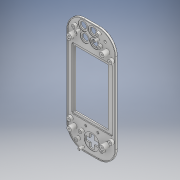
# Autodesk Inventor part: Partie Haute
Saved by Autodesk Inventor 2019 (Build 230136000, 136)
## iProperties
Created: 2018-06-04
Part Number: Partie Haute
Material: Plastique ABS
Document SubType Name: Modeling
Designer: dimercur
Mass: 33.4768 g
Surface Area: 274.719 cm^2
Volume: 31.5819 cm^3
Density: 1.06 g/cm^3
Appearance: Lisse - Blanc
Author: dimercur
Autodesk Inventor part; units mm, degrees
ref_plane "YZ Plane" through (0, 0, 0) normal (1, 0, 0) x (0, 1, 0)
ref_plane "XZ Plane" through (0, 0, 0) normal (0, 1, 0) x (-1, 0, 0)
ref_plane "XY Plane" through (0, 0, 0) normal (0, 0, 1) x (1, 0, 0)
sketch "Esquisse1" plane through (0, 0, 0) normal (0, 1, 0) x (-1, 0, 0)
  line L0 (42.5, 100) -> (-42.5, 100)
  line L1 (-42.5, 100) -> (-42.5, -100)
  line L2 (-42.5, -100) -> (42.5, -100)
  line L3 (42.5, -100) -> (42.5, 100)
  point P0 (0, 0)
  dimension "d0" = 200
  dimension "d1" = 85
  dimension "d2" = 42.5
  dimension "d3" = 100
  constraints: 8 end point, 2 parallel, 1 horizontal, 1 perpendicular
  measures "d0" distance of L2.end L0.start
  measures "d1" distance of L0.start L0.end
  measures "d2" horizontal distance of point (0, 0) L0.start
  measures "d3" vertical distance of point (0, 0) L0.start
extrude "Extrusion1" add sketch "Esquisse1" along normal blind 42
chamfer "Chanfrein1" distance 20 angle 60 1 edges at (0, 0, 100) measured on face at (0, 0.5, 100)
chamfer "Chanfrein2" distance 20 angle 60 1 edges at (0, 0, -100) measured on face at (0, 0.5, -100)
fillet "Congé3" radius 30 4 edges at (-42.5, 31, 100) (42.5, 31, 100) (-42.5, 31, -100) (42.5, 31, -100)
fillet "Congé4" radius 15 14 edges at (0, 0, 65.359) (-33.7132, 14.9269, 91.2132) (-42.5, 1.3397, 67.6795) (33.7132, 14.9269, 91.2132) (42.5, 1.3397, 67.6795) (0, 20, 100) (-42.5, 0, 0) (42.5, 0, 0) (0, 0, -65.359) (33.7132, 14.9269, -91.2132) (42.5, 1.3397, -67.6795) (-33.7132, 14.9269, -91.2132) (-42.5, 1.3397, -67.6795) (0, 20, -100)
shell "Coque1" thickness 2.5 removed faces 1 at (-14.1667, 42, -23.3333)
sketch "Esquisse3" plane through (0, 42, 0) normal (0, 1, 0) x (1, 0, 0)
  arc A0 (42.5, 70) -> (12.5, 100) centre (12.5, 70) ccw projected
  line L0 (12.5, 100) -> (-12.5, 100) projected
  arc A1 (-12.5, 100) -> (-42.5, 70) centre (-12.5, 70) ccw projected
  line L1 (-42.5, 70) -> (-42.5, -70) projected
  arc A2 (-42.5, -70) -> (-12.5, -100) centre (-12.5, -70) ccw projected
  line L2 (-12.5, -100) -> (12.5, -100) projected
  arc A3 (12.5, -100) -> (42.5, -70) centre (12.5, -70) ccw projected
  line L3 (42.5, -70) -> (42.5, 70) projected
  point P0 (0, 0)
extrude "Extrusion2" add sketch "Esquisse3" along normal blind 2.5
sketch "Esquisse4" plane through (0, 44.5, 0) normal (0, 1, 0) x (1, 0, 0)
  line L0 (36.5, 54) -> (-34.5, 54)
  line L1 (-34.5, 54) -> (-34.5, -54)
  line L2 (-34.5, -54) -> (36.5, -54)
  line L3 (36.5, -54) -> (36.5, 54)
  line L4 (27.5, -67.5897) -> (-27.5, -67.5897) projected
  line L5 (42.5, -70) -> (42.5, 70) projected
  line L6 (-42.5, 70) -> (-42.5, -70) projected
  line L7 (12.5, 100) -> (-12.5, 100) projected
  line L8 (-12.5, -100) -> (12.5, -100) projected
  point P0 (0, 0)
  dimension "d19" = 108
  dimension "d20" = 71
  dimension "d21" = 36.5
  dimension "d22" = 54
  dimension "d154" = 85
  dimension "d155" = 46
  constraints: 8 end point, 2 parallel, 1 horizontal, 1 perpendicular
  measures "d19" distance of L2.end L0.start
  measures "d20" distance of L0.start L0.end
  measures "d21" horizontal distance of point (0, 0) L0.start
  measures "d22" vertical distance of point (0, 0) L0.start
  measures "d154" distance between parallel lines of L6 L5
  measures "d155" distance between parallel lines of L8 L2
extrude "Extrusion15" cut sketch "Esquisse4" against normal through all
sketch "Esquisse5" plane through (-40, 15, 61.3397) normal (1, 0, 0) x (0, 0, -1)
  line L0 (-48.6603, 26) -> (171.3397, 26)
  line L1 (171.3397, 26) -> (171.3397, -24)
  line L2 (171.3397, -24) -> (-48.6603, -24)
  line L3 (-48.6603, -24) -> (-48.6603, 26)
  line L4 (-36.1603, 27) -> (-8.6603, 27) projected
  line L5 (-38.6603, 29.5) -> (-38.6603, 13.6603) projected
  line L6 (161.3397, 13.6603) -> (161.3397, 29.5) projected
  point P0 (61.3397, -15)
  dimension "d47" = 1
  dimension "d48" = 220
  dimension "d50" = 200
  dimension "d51" = 10
  dimension "d52" = 50
  constraints: 8 end point, 2 parallel, 1 horizontal, 1 perpendicular
  measures "d47" distance between parallel lines of L4 L0
  measures "d48" distance between parallel lines of L1 L3
  measures "d50" distance between parallel lines of L6 L5
  measures "d51" distance between parallel lines of L5 L3
  measures "d52" distance between parallel lines of L0 L2
extrude "Extrusion4" cut sketch "Esquisse5" along normal through all both and the other way through all
sketch "Esquisse6" plane through (-12.5, 41, -100) normal (0, -1, 0) x (1, 0, 0)
  line L0 (-27.5, 170) -> (-27.5, 30) projected
  arc A0 (-27.5, 30) -> (0, 2.5) centre (0, 30) ccw projected
  line L1 (0, 2.5) -> (25, 2.5) projected
  arc A1 (25, 2.5) -> (52.5, 30) centre (25, 30) ccw projected
  line L2 (52.5, 30) -> (52.5, 170) projected
  arc A2 (52.5, 170) -> (25, 197.5) centre (25, 170) ccw projected
  line L3 (25, 197.5) -> (0, 197.5) projected
  arc A3 (0, 197.5) -> (-27.5, 170) centre (0, 170) ccw projected
  line L4 (-28.75, 30) -> (-28.75, 170)
  arc A4 (0, 198.75) -> (-28.75, 170) centre (0, 170) ccw
  line L5 (0, 198.75) -> (25, 198.75)
  arc A5 (53.75, 170) -> (25, 198.75) centre (25, 170) ccw
  line L6 (53.75, 170) -> (53.75, 30)
  arc A6 (25, 1.25) -> (53.75, 30) centre (25, 30) ccw
  line L7 (25, 1.25) -> (0, 1.25)
  arc A7 (-28.75, 30) -> (0, 1.25) centre (0, 30) ccw
  line L8 (-30, 30) -> (-30, 170) projected
  point P0 (12.5, 100)
  dimension "d55" = 2.5
  dimension "d56" = 1.25
  constraints: 8 end point, 8 point on circle, 4 centre point, 7 other
  measures "d55" distance between parallel lines of L0 L8
  measures "d56" distance between parallel lines of L0 L4
extrude "Extrusion5" cut sketch "Esquisse6" against normal blind 1
sketch "Esquisse7" plane through (0, 42, 0) normal (0, -1, 0) x (1, 0, 0)
  circle A0 centre (-36, -61) radius 3.75
  circle A1 centre (36, -61) radius 3.75
  circle A2 centre (36, 61) radius 3.75
  circle A3 centre (-36, 61) radius 3.75
  point P0 (0, 0)
  dimension "d59" = 7.5
  dimension "d60" = 7.5
  dimension "d61" = 7.5
  dimension "d62" = 7.5
  dimension "d63" = 122
  dimension "d64" = 72
  dimension "d65" = 122
  dimension "d66" = 72
  dimension "d67" = 61
  dimension "d68" = 36
  dimension "d69" = 36
  dimension "d70" = 61
  constraints: 4 centre point
  measures "d59" diameter of A0
  measures "d60" diameter of A1
  measures "d61" diameter of A2
  measures "d62" diameter of A3
  measures "d63" distance of A3.centre A0.centre
  measures "d64" distance of A1.centre A0.centre
  measures "d65" distance of A2.centre A1.centre
  measures "d66" distance of A2.centre A3.centre
  measures "d67" vertical distance of point (0, 0) A0.centre
  measures "d68" horizontal distance of point (0, 0) A3.centre
  measures "d69" horizontal distance of point (0, 0) A0.centre
  measures "d70" vertical distance of point (0, 0) A1.centre
extrude "Extrusion6" add sketch "Esquisse7" along normal blind 4.5
sketch "Esquisse8" plane through (-36, 37.5, -61) normal (0, -1, 0) x (1, 0, 0)
  circle A0 centre (0, 0) radius 1.2
  circle A1 centre (0, 122) radius 1.2
  circle A2 centre (72, 122) radius 1.2
  circle A3 centre (72, 0) radius 1.2
  circle A4 centre (72, 122) radius 3.75 projected
  circle A5 centre (0, 122) radius 3.75 projected
  circle A6 centre (0, 0) radius 3.75 projected
  point P0 (36, 61)
  dimension "d73" = 2.4
  dimension "d74" = 2.4
  dimension "d75" = 2.4
  dimension "d76" = 2.4
  dimension "d77" = 72
  dimension "d78" = 122
  dimension "d79" = 122
  dimension "d80" = 72
  dimension "d81" = 122
  dimension "d82" = 72
  dimension "d83" = 61
  dimension "d84" = 61
  dimension "d85" = 36
  dimension "d86" = 36
  constraints: 4 centre point
  measures "d73" diameter of A0
  measures "d74" diameter of A1
  measures "d75" diameter of A2
  measures "d76" diameter of A3
  measures "d77" distance of A4.centre A5.centre
  measures "d78" distance of A5.centre A6.centre
  measures "d79" distance of A1.centre A0.centre
  measures "d80" distance of A2.centre A1.centre
  measures "d81" distance of A3.centre A2.centre
  measures "d82" distance of A3.centre A0.centre
  measures "d83" vertical distance of point (36, 61) A3.centre
  measures "d84" vertical distance of point (36, 61) A0.centre
  measures "d85" horizontal distance of point (36, 61) A0.centre
  measures "d86" horizontal distance of point (36, 61) A1.centre
extrude "Extrusion7" cut sketch "Esquisse8" against normal blind 5 contours A0 | A1 | A2 | A3
fillet "Congé6" radius 0.5 8 edges at (33.7132, 44.5, -91.2132) (0, 44.5, -100) (-33.7132, 44.5, -91.2132) (-42.5, 44.5, 0) (-33.7132, 44.5, 91.2132) (0, 44.5, 100) (33.7132, 44.5, 91.2132) (42.5, 44.5, 0)
sketch "Esquisse11" plane through (0, 42, 0) normal (0, -1, 0) x (1, 0, 0)
  circle A0 centre (-29.5, -70) radius 4
  circle A1 centre (27.5, -70) radius 4
  circle A2 centre (27.5, 70) radius 4
  circle A3 centre (-29.5, 70) radius 4
  line L0 (-42.5, -70) -> (-42.5, 70) projected
  line L1 (42.5, 70) -> (42.5, -70) projected
  line L2 (12.5, -100) -> (-12.5, -100) projected
  line L3 (-12.5, 100) -> (12.5, 100) projected
  circle A4 centre (-29.5, -70) radius 1.25
  circle A5 centre (27.5, -70) radius 1.25
  circle A6 centre (27.5, 70) radius 1.25
  circle A7 centre (-29.5, 70) radius 1.25
  point P0 (0, 0)
  dimension "d134" = 8
  dimension "d135" = 8
  dimension "d136" = 8
  dimension "d137" = 8
  dimension "d138" = 13
  dimension "d139" = 15
  dimension "d140" = 15
  dimension "d141" = 13
  dimension "d142" = 30
  dimension "d143" = 30
  dimension "d144" = 30
  dimension "d145" = 30
  dimension "d146" = 2.5
  dimension "d147" = 2.5
  dimension "d148" = 2.5
  dimension "d149" = 2.5
  constraints: 8 centre point, 4 coincident
  measures "d134" diameter of A0
  measures "d135" diameter of A1
  measures "d136" diameter of A3
  measures "d137" diameter of A2
  measures "d138" distance from line of L0 A0.centre
  measures "d139" distance from line of L1 A1.centre
  measures "d140" distance from line of L1 A2.centre
  measures "d141" distance from line of L0 A3.centre
  measures "d142" distance from line of A0.centre L2
  measures "d143" distance from line of L2 A1.centre
  measures "d144" distance from line of L3 A2.centre
  measures "d145" distance from line of L3 A3.centre
  measures "d146" diameter of A4
  measures "d147" diameter of A5
  measures "d148" diameter of A7
  measures "d149" diameter of A6
extrude "Extrusion10" add sketch "Esquisse11" along normal blind 10
sketch "Esquisse15" plane through (0, 44.5, 0) normal (0, 1, 0) x (1, 0, 0)
  circle A0 centre (10.5, 62) radius 0.75
  line L0 (-34.5, 54) -> (36.5, 54) projected
  line L1 (42.5, -70) -> (42.5, 70) projected
  circle A1 centre (10.5, 59) radius 0.75
  circle A2 centre (12, 60.5) radius 0.75
  circle A3 centre (9, 60.5) radius 0.75
  circle A4 centre (-10.5, 62) radius 0.75
  circle A5 centre (-10.5, 59) radius 0.75
  circle A6 centre (-9, 60.5) radius 0.75
  circle A7 centre (-12, 60.5) radius 0.75
  point P0 (0, 0)
  dimension "d189" = 1.5
  dimension "d190" = 8
  dimension "d191" = 32
  dimension "d192" = 1.5
  dimension "d193" = 1.5
  dimension "d194" = 1.5
  dimension "d195" = 32
  dimension "d196" = 5
  dimension "d197" = 6.5
  dimension "d198" = 6.5
  dimension "d199" = 3
  dimension "d200" = 3
  dimension "d201" = 30.5
  dimension "d204" = 21
  constraints: 8 centre point, 1 horizontal, 8 other
  measures "d189" diameter of A0
  measures "d190" distance from line of L0 A0.centre
  measures "d191" distance from line of L1 A0.centre
  measures "d192" diameter of A2
  measures "d193" diameter of A1
  measures "d194" diameter of A3
  measures "d195" distance from line of L1 A1.centre
  measures "d196" distance from line of L0 A1.centre
  measures "d197" distance from line of L0 A2.centre
  measures "d198" distance from line of L0 A3.centre
  measures "d199" distance of A0.centre A1.centre
  measures "d200" distance of A3.centre A2.centre
  measures "d201" distance from line of L1 A2.centre
  measures "d204" distance of A0.centre A4.centre
extrude "Extrusion13" cut sketch "Esquisse15" against normal through all
sketch "Esquisse16" plane through (0, 44.5, 0) normal (0, 1, 0) x (1, 0, 0)
  line L0 (40, 57.5) -> (-38, 57.5)
  line L1 (-38, 57.5) -> (-38, -57.5)
  line L2 (-38, -57.5) -> (40, -57.5)
  line L3 (40, -57.5) -> (40, 57.5)
  line L4 (27, 49.5) -> (-31, 49.5)
  line L5 (-31, 49.5) -> (-31, -49.5)
  line L6 (-31, -49.5) -> (27, -49.5)
  line L7 (27, -49.5) -> (27, 49.5)
  line L8 (36.5, 54) -> (36.5, -54) projected
  line L9 (-34.5, 54) -> (36.5, 54) projected
  line L10 (36.5, -54) -> (-34.5, -54) projected
  line L11 (-34.5, -54) -> (-34.5, 54) projected
  point P0 (0, 0)
  dimension "d211" = 99
  dimension "d212" = 49.5
  dimension "d213" = 78
  dimension "d215" = 3.5
  dimension "d217" = 3.5
  dimension "d218" = 3.5
  dimension "d219" = 58
  dimension "d225" = 3.5
  constraints: 16 end point, 4 parallel, 2 horizontal, 2 perpendicular
  measures "d211" distance of L6.end L4.start
  measures "d212" vertical distance of point (0, 0) L4.start
  measures "d213" distance of L0.start L0.end
  measures "d215" distance between parallel lines of L8 L3
  measures "d217" distance between parallel lines of L9 L0
  measures "d218" distance between parallel lines of L10 L2
  measures "d219" distance of L4.start L4.end
  measures "d225" distance between parallel lines of L11 L5
extrude "Extrusion14" add sketch "Esquisse16" along normal blind 1.5 and the other way blind 1 contours L3 L2 L1 L0 | L8 L10 L11 L9
chamfer "Chanfrein4" distance 0.5 angle 45 4 edges at (27, 46, 0) (-2, 46, -49.5) (-2, 46, 49.5) (-31, 46, 0)
fillet "Congé14" radius 8 4 edges at (-38, 45.25, -57.5) (-38, 45.25, 57.5) (40, 45.25, 57.5) (40, 45.25, -57.5)
fillet "Congé15" radius 0.5 16 edges at (37.6569, 44.5, -55.1569) (40, 44.5, 0) (37.6569, 44.5, 55.1569) (1, 44.5, 57.5) (-35.6569, 44.5, 55.1569) (-38, 44.5, 0) (-35.6569, 44.5, -55.1569) (1, 44.5, -57.5) (1, 46, -57.5) (37.6569, 46, -55.1569) (40, 46, 0) (37.6569, 46, 55.1569) (1, 46, 57.5) (-35.6569, 46, 55.1569) (-38, 46, 0) (-35.6569, 46, -55.1569)
fillet "Congé16" radius 3 4 edges at (36.5, 42.75, -54) (-34.5, 42.75, -54) (-34.5, 42.75, 54) (36.5, 42.75, 54)
fillet "Congé17" radius 0.5 8 edges at (35.6213, 43.5, -53.1213) (1, 43.5, -54) (-33.6213, 43.5, -53.1213) (-34.5, 43.5, 0) (-33.6213, 43.5, 53.1213) (1, 43.5, 54) (35.6213, 43.5, 53.1213) (36.5, 43.5, 0)
sketch "Esquisse9" plane through (0, 44.5, 0) normal (0, 1, 0) x (1, 0, 0)
  line L0 (10.75, 83) -> (-10.75, 83)
  line L1 (-10.75, 83) -> (-10.75, 75.5)
  line L2 (-10.75, 75.5) -> (10.75, 75.5)
  line L3 (10.75, 75.5) -> (10.75, 83)
  line L4 (3.75, 90) -> (-3.75, 90)
  line L5 (-3.75, 90) -> (-3.75, 68.5)
  line L6 (-3.75, 68.5) -> (3.75, 68.5)
  line L7 (3.75, 68.5) -> (3.75, 90)
  line L8 (12.5, 100) -> (-12.5, 100) projected
  line L9 (-42.5, 70) -> (-42.5, -70) projected
  line L10 (42.5, -70) -> (42.5, 70) projected
  point P0 (0, 0)
  dimension "d98" = 21.5
  dimension "d99" = 21.5
  dimension "d100" = 7.5
  dimension "d101" = 7.5
  dimension "d102" = 7
  dimension "d103" = 7
  dimension "d104" = 10
  dimension "d105" = 31.75
  dimension "d156" = 85
  constraints: 16 end point, 4 parallel, 2 horizontal, 2 perpendicular
  measures "d98" distance of L6.end L4.start
  measures "d99" distance of L0.start L0.end
  measures "d100" distance of L4.start L4.end
  measures "d101" distance of L2.end L0.start
  measures "d102" distance between parallel lines of L3 L7
  measures "d103" distance from line of L0 L4.start
  measures "d104" distance between parallel lines of L8 L4
  measures "d105" distance between parallel lines of L9 L1
  measures "d156" distance between parallel lines of L9 L10
extrude "Extrusion8" cut sketch "Esquisse9" against normal through all
sketch "Esquisse14" plane through (0, 44.5, 0) normal (0, 1, 0) x (1, 0, 0)
  circle A0 centre (23.25, -83) radius 2.1
  line L0 (-12.5, -100) -> (12.5, -100) projected
  line L1 (42.5, -70) -> (42.5, 70) projected
  circle A1 centre (2, -88) radius 5.5
  circle A2 centre (5, -71.2668) radius 5.5
  circle A3 centre (-12, -71.2668) radius 5.5
  circle A4 centre (-15, -88) radius 5.5
  point P0 (0, 0)
  dimension "d184" = 4.2
  dimension "d185" = 17
  dimension "d186" = 19.25
  dimension "d241" = 11
  dimension "d242" = 11
  dimension "d243" = 11
  dimension "d244" = 11
  dimension "d245" = 17
  dimension "d246" = 17
  dimension "d247" = 28
  dimension "d248" = 28
  dimension "d249" = 2
  dimension "d250" = 12
  dimension "d251" = 12
  dimension "d252" = 5
  constraints: 5 centre point
  measures "d184" diameter of A0
  measures "d185" distance from line of L0 A0.centre
  measures "d186" distance from line of L1 A0.centre
  measures "d241" diameter of A2
  measures "d242" diameter of A1
  measures "d243" diameter of A3
  measures "d244" diameter of A4
  measures "d245" distance of A4.centre A1.centre
  measures "d246" distance of A3.centre A2.centre
  measures "d249" horizontal distance of point (0, 0) A1.centre
  measures "d250" distance from line of L0 A1.centre
  measures "d251" distance from line of L0 A4.centre
  measures "d252" horizontal distance of point (0, 0) A2.centre
extrude "Extrusion12" cut sketch "Esquisse14" against normal through all
sketch "Esquisse12" plane through (0, 42, 0) normal (0, -1, 0) x (1, 0, 0)
  circle A0 centre (21.5, -81.5) radius 3
  circle A1 centre (-22.5, -85) radius 3
  line L0 (12.5, -98.75) -> (-12.5, -98.75) projected
  line L1 (-41.25, -70) -> (-41.25, 70) projected
  line L2 (41.25, 70) -> (41.25, -70) projected
  circle A2 centre (-22.5, -85) radius 1
  circle A3 centre (21.5, -81.5) radius 1
  line L3 (-12.5, 98.75) -> (12.5, 98.75) projected
  circle A4 centre (-16, -70) radius 3
  circle A5 centre (-16, -70) radius 1
  line L4 (-42.5, -70) -> (-42.5, 70) projected
  line L5 (42.5, 70) -> (42.5, -70) projected
  line L6 (12.5, -100) -> (-12.5, -100) projected
  point P0 (0, 0)
  dimension "d157" = 6
  dimension "d158" = 6
  dimension "d166" = 2
  dimension "d167" = 2
  dimension "d288" = 6
  dimension "d289" = 2
  dimension "d306" = 26.5
  dimension "d307" = 20
  dimension "d308" = 21
  dimension "d309" = 18.5
  dimension "d310" = 15
  dimension "d311" = 30
  constraints: 6 centre point, 3 coincident
  measures "d157" diameter of A1
  measures "d158" diameter of A0
  measures "d166" diameter of A2
  measures "d167" diameter of A3
  measures "d288" diameter of A4
  measures "d289" diameter of A5
  measures "d306" distance from line of A4.centre L4
  measures "d307" distance from line of A2.centre L4
  measures "d308" distance from line of A0.centre L5
  measures "d309" distance from line of L6 A0.centre
  measures "d310" distance from line of A1.centre L6
  measures "d311" distance from line of L6 A4.centre
extrude "Extrusion11" add sketch "Esquisse12" along normal blind 4.7
sketch "Esquisse17" plane through (0, 42, 0) normal (0, -1, 0) x (1, 0, 0)
  circle A0 centre (-14.769, -94.179) radius 2
  line L0 (3.75, -90) -> (-3.75, -90) projected
  line L1 (-3.75, -90) -> (-3.75, -83) projected
  point P0 (0, 0)
  dimension "d253" = 4
  dimension "d254" = 4.179
  dimension "d255" = 11.019
  constraints: 1 centre point
  measures "d253" diameter of A0
  measures "d254" distance from line of A0.centre L0
  measures "d255" distance from line of A0.centre L1
extrude "Extrusion16" add sketch "Esquisse17" along normal blind 8
chamfer "Chanfrein5" distance 0.5 angle 45 1 edges at (-16.769, 34, -94.179)
sketch "Esquisse18" plane through (0, 42, 0) normal (0, -1, 0) x (1, 0, 0)
  circle A0 centre (0, -79.25) radius 13.5
  line L0 (3.75, -90) -> (-3.75, -90) projected
  line L1 (-3.75, -68.5) -> (3.75, -68.5) projected
  line L2 (-10.75, -83) -> (-10.75, -75.5) projected
  point P0 (0, 0)
  dimension "d265" = 27
  dimension "d266" = 21.5
  dimension "d267" = 10.75
  dimension "d268" = 10.75
  constraints: 1 centre point
  measures "d265" diameter of A0
  measures "d266" distance between parallel lines of L0 L1
  measures "d267" distance from line of L0 A0.centre
  measures "d268" distance from line of A0.centre L2
extrude "Extrusion17" cut sketch "Esquisse18" against normal blind 0.5
sketch "Esquisse19" plane through (0, 42, 0) normal (0, -1, 0) x (1, 0, 0)
  circle A0 centre (-12, 71.2668) radius 8.25
  circle A1 centre (-15, 88) radius 8.25
  circle A2 centre (2, 88) radius 8.25
  circle A3 centre (5, 71.2668) radius 8.25
  circle A4 centre (-12, 71.2668) radius 5.5 projected
  circle A5 centre (-15, 88) radius 5.5 projected
  circle A6 centre (2, 88) radius 5.5 projected
  circle A7 centre (5, 71.2668) radius 5.5 projected
  point P0 (0, 0)
  dimension "d271" = 16.5
  dimension "d272" = 16.5
  dimension "d273" = 16.5
  dimension "d274" = 16.5
  constraints: 4 centre point, 4 concentric
  measures "d271" diameter of A0
  measures "d272" diameter of A1
  measures "d273" diameter of A2
  measures "d274" diameter of A3
extrude "Extrusion18" cut sketch "Esquisse19" against normal blind 0.5
sketch "Esquisse20" plane through (0, 42, 0) normal (0, -1, 0) x (1, 0, 0)
  circle A0 centre (-21.178, 78.5608) radius 2
  circle A1 centre (11.178, 80.706) radius 2
  circle A2 centre (2, 88) radius 5.5 projected
  circle A3 centre (-12, 71.2668) radius 5.5 projected
  point P0 (0, 0)
  dimension "d277" = 4
  dimension "d278" = 4
  dimension "d279" = 9.178
  dimension "d280" = 7.294
  dimension "d281" = 9.178
  dimension "d282" = 7.294
  constraints: 2 centre point
  measures "d277" diameter of A0
  measures "d278" diameter of A1
  measures "d279" horizontal distance of A1.centre A2.centre
  measures "d280" vertical distance of A1.centre A2.centre
  measures "d281" horizontal distance of A3.centre A0.centre
  measures "d282" vertical distance of A0.centre A3.centre
extrude "Extrusion19" add sketch "Esquisse20" along normal blind 7 contours A0 | A1
chamfer "Chanfrein6" distance 0.5 angle 45 2 edges at (-23.178, 35, 78.5608) (9.178, 35, 80.706)
sketch "Esquisse21" plane through (0, 42, 0) normal (0, -1, 0) x (1, 0, 0)
  circle A0 centre (-27.5, 83) radius 3
  circle A1 centre (-27.5, 83) radius 1
  circle A2 centre (16.5, 73) radius 3
  circle A3 centre (16.5, 73) radius 1
  circle A4 centre (13.5, 91) radius 3
  circle A5 centre (13.5, 91) radius 1
  line L0 (-12.5, 98.75) -> (12.5, 98.75) projected
  line L1 (-41.25, -70) -> (-41.25, 70) projected
  line L2 (-42.5, -70) -> (-42.5, 70) projected
  line L3 (-12.5, 100) -> (12.5, 100) projected
  point P0 (0, 0)
  dimension "d292" = 6
  dimension "d293" = 6
  dimension "d294" = 6
  dimension "d295" = 2
  dimension "d296" = 2
  dimension "d297" = 2
  dimension "d312" = 15
  dimension "d313" = 56
  dimension "d314" = 59
  dimension "d315" = 17
  dimension "d316" = 9
  dimension "d317" = 27
  constraints: 6 centre point, 3 coincident
  measures "d292" diameter of A0
  measures "d293" diameter of A4
  measures "d294" diameter of A2
  measures "d295" diameter of A1
  measures "d296" diameter of A5
  measures "d297" diameter of A3
  measures "d312" distance from line of A0.centre L2
  measures "d313" distance from line of A4.centre L2
  measures "d314" distance from line of A2.centre L2
  measures "d315" distance from line of A0.centre L3
  measures "d316" distance from line of L3 A4.centre
  measures "d317" distance from line of L3 A2.centre
extrude "Extrusion20" add sketch "Esquisse21" along normal blind 4.7
equation "\"d2\" = 0.5 * d1"
equation "\"d3\" = 0.5 * d0"
equation "\"d22\" = 0.5 * d19"
equation "\"d51\" = -0.5 * d50 + 0.5 * d48"
equation "\"d56\" = 0.5 * d55"
equation "\"d60\" = d59"
equation "\"d61\" = d59"
equation "\"d62\" = d59"
equation "\"d65\" = d63"
equation "\"d66\" = d64"
equation "\"d67\" = 0.5 * d63"
equation "\"d68\" = 0.5 * d66"
equation "\"d69\" = 0.5 * d64"
equation "\"d70\" = 0.5 * d63"
equation "\"d74\" = d73"
equation "\"d75\" = d73"
equation "\"d76\" = d73"
equation "\"d79\" = d78"
equation "\"d80\" = d77"
equation "\"d81\" = d78"
equation "\"d82\" = d77"
equation "\"d83\" = 0.5 * d78"
equation "\"d84\" = 0.5 * d78"
equation "\"d85\" = 0.5 * d77"
equation "\"d86\" = 0.5 * d77"
equation "\"d135\" = d134"
equation "\"d136\" = d134"
equation "\"d137\" = d134"
equation "\"d140\" = d139"
equation "\"d141\" = d138"
equation "\"d143\" = d142"
equation "\"d144\" = d143"
equation "\"d145\" = d142"
equation "\"d147\" = d146"
equation "\"d148\" = d146"
equation "\"d149\" = d146"
equation "\"d192\" = d189"
equation "\"d193\" = d189"
equation "\"d194\" = d189"
equation "\"d198\" = d197"
equation "\"d200\" = d199"
equation "\"d212\" = 0.5 * d211"
equation "\"d217\" = d215"
equation "\"d218\" = d215"
equation "\"d99\" = d98"
equation "\"d101\" = d100"
equation "\"d102\" = -0.5 * d100 + 0.5 * d98"
equation "\"d103\" = -0.5 * d100 + 0.5 * d98"
equation "\"d105\" = 0.5 * d156 - 0.5 * d98"
equation "\"d158\" = d157"
equation "\"d167\" = d166"
